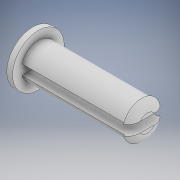
# Autodesk Inventor part: OsovinaZaPrednjiKotač_v.1.0
Saved by Autodesk Inventor 2020 (Build 240168000, 168)
## iProperties
Created: 2020-10-16
Part Number: OsovinaZaPrednjiKotač_v.1.0
Material: Generic
Document SubType Name: Modeling
Designer: Sičaja
Density: 1 g/cm^3
Appearance: Default
Author: Sičaja
Autodesk Inventor part; units mm, degrees
ref_plane "YZ Plane" through (0, 0, 0) normal (1, 0, 0) x (0, 1, 0)
ref_plane "XZ Plane" through (0, 0, 0) normal (0, 1, 0) x (-1, 0, 0)
ref_plane "XY Plane" through (0, 0, 0) normal (0, 0, 1) x (1, 0, 0)
sketch "Sketch1" plane through (0, 0, 0) normal (1, 0, 0) x (0, 1, 0)
  circle A0 centre (0, 0) radius 3
  dimension "d0" = 6
  constraints: 1 centre point, 1 coincident
  measures "d0" diameter of A0
extrude "Extrusion1" add sketch "Sketch1" along normal mid plane 18
sketch "Sketch2" plane through (-9, 0, 0) normal (-1, 0, 0) x (0, 0, 1)
  circle A0 centre (0, 0) radius 4.5
  dimension "d3" = 9
  constraints: 1 centre point, 1 coincident
  measures "d3" diameter of A0
extrude "Extrusion2" add sketch "Sketch2" along normal blind 1
sketch "Sketch3" plane through (9, 0, 0) normal (1, 0, 0) x (0, 0, -1)
  circle A0 centre (0, 0) radius 3.25
  dimension "d6" = 6.5
  constraints: 1 centre point, 1 coincident
  measures "d6" diameter of A0
extrude "Extrusion3" add sketch "Sketch3" along normal blind 1
sketch "Sketch4" plane through (10, 0, 0) normal (1, 0, 0) x (0, 0, -1)
  circle A0 centre (0, 0) radius 3.25 projected
  line L0 (-3.1282, 0.8815) -> (3.1282, 0.8815)
  line L1 (-3.25, 0) -> (3.25, 0)
  line L2 (-3.1282, -0.8815) -> (3.1282, -0.8815)
  arc A1 (-3.1282, 0.8815) -> (-3.1282, -0.8815) centre (0, 0) ccw
  arc A2 (3.1282, -0.8815) -> (3.1282, 0.8815) centre (0, 0) ccw
  constraints: 8 point on circle, 6 end point, 2 centre point, 2 symmetric about line, 1 coincident, 1 horizontal, 1 parallel
extrude "Extrusion4" cut sketch "Sketch4" against normal blind 19 contours L1 A0 L0 | A0 L2 L1
fillet "Fillet1" radius 2 2 edges at (10, 3.25, 0) (10, -3.25, 0)
body "Solid1"
